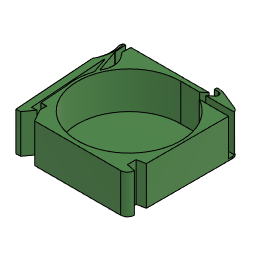
Compliant Strip Holder v3 (Autodesk Fusion 360 design; units mm, degrees)
Autodesk Fusion 360 part; units mm, degrees
sketch "Sketch1" plane through (0, 0, 0) normal (0, 0, 1) x (1, 0, 0) in component "Compliant SMD Magazine"
  line L0 (26.5, 5) -> (26.5, 10)
  line L1 (26.5, 10) -> (31.5, 11)
  line L2 (31.5, 4) -> (26.5, 5)
  line L3 (26.5, 7.5) -> (31.5, 7.5) construction
  line L4 (31.5, 4) -> (31.5, 0)
  line L5 (31.5, 0) -> (-22.4585, 0)
  line L6 (-22.4585, 0) -> (-26.5, 7)
  line L7 (-26.5, 7) -> (-26.5, 11)
  line L8 (-26.5, 11) -> (-31.5, 11)
  line L9 (31.5, 11) -> (31.5, 4) construction
  line L10 (31.5, 11) -> (31.5, 65)
  line L11 (31.5, 65) -> (-31.5, 65)
  circle A0 centre (0, 32.5) radius 30
  line L12 (0, 0) -> (0, 65) construction
  line L13 (-31.5, 65) -> (-31.5, 11)
  line L14 (30, 32.5) -> (-30, 32.5) construction
  line L15 (0, 1.75) -> (0, 22.5)
  point P0 (-30, 32.5)
  dimension "d28" = 5
  dimension "d29" = 7
  dimension "d30" = 58
  dimension "d31" = 4
  dimension "d32" = 4
  dimension "d34" = 120
  dimension "d36" = 11
  dimension "d37" = 5
  dimension "d38" = 54
  dimension "d39" = 60
  dimension "d43" = 1.5
  dimension "d44" = 1.5
  constraint midpoint L3.start L0
  constraint symmetric L1 L2 L3
  constraint vertical L4
  constraint perpendicular L4 L5
  constraint perpendicular L5 L7
  constraint perpendicular L7 L8
  constraint vertical L0
  constraint equal L1 L2
  constraint coincident L3.end L9
  constraint coincident L12.start L5
  constraint parallel L9 L10
  constraint perpendicular L10 L11
  constraint coincident L5 L12.start
  constraint coincident L11 L12.end
  constraint perpendicular L11 L12
  constraint midpoint A0.centre L12
  constraint vertical L13
  constraint coincident A0 L14.start
  constraint coincident A0 P0
  constraint horizontal L14
  constraint coincident A0.centre L14
  constraint coincident P0 L14.end
  constraint coincident A0.centre L15
  measures "d28" distance of L0.start L0.end
  measures "d29" distance of L2.start L1.end
  measures "d30" distance of L4 L7
  measures "d31" distance of L2.start L4.end
  measures "d32" distance of L6.end L7.end
  measures "d34" angle of L5 L6
  measures "d36" distance of L5 L8
  measures "d37" horizontal distance of L2.start L0.start
  measures "d38" distance of L1.end L10.end
  measures "d39" diameter of A0
  measures "d43" distance of L13 P0
  measures "d44" distance of L10 L14.start
extrude "Extrude1" add sketch "Sketch1" against normal blind 1 contours L0 L1 L2 L4 L5 L6 L7 L8 L10 L11 L13 | A0 makes body 1 in component "Compliant SMD Magazine"
extrude "Extrude2" add sketch "Sketch1" along normal blind 21.5 bodies 1 in component "Compliant SMD Magazine"
sketch "Sketch2" plane through (0, 0, 21.5) normal (0, 0, 1) x (-1, 0, 0) in component "Compliant SMD Magazine"
  circle A0 centre (0, -32.5) radius 30
  line L0 (-31.5, -11) -> (-31.5, -65)
  line L1 (-31.5, -65) -> (31.5, -65)
  line L2 (-14.5237, -58.75) -> (-31.5, -58.75)
  line L3 (0, -62.5) -> (-31.5, -62.5)
  line L4 (-10.996, -62.5) -> (-14, -65)
  line L5 (-14.496, -62.5) -> (-17.5, -65)
  dimension "d53" = 3.75
  dimension "d77" = 14
  dimension "d78" = 3.5
  constraint coincident A0 L2.start
  constraint coincident L0 L2.end
  constraint perpendicular L0 L2
  constraint coincident A0 L3.start
  constraint coincident L0 L3.end
  constraint perpendicular L0 L3
  constraint tangent A0 L3
  constraint coincident L3 L4.start
  constraint coincident L1 L4.end
  constraint coincident L3 L5.start
  constraint coincident L1 L5.end
  constraint parallel L4 L5
  measures "d53" distance of L2 L3
  measures "d77" distance of L0.end L5.end
  measures "d78" distance of L4.end L5.end
extrude "Extrude3" cut sketch "Sketch2" against normal blind 21.5 contours A0 L0 L2 L3 | L1 L3 L4 L5 bodies 1 in component "Compliant SMD Magazine"
fillet "Fillet1" radius 4 1 edges at (31.5, 65, 10.25) on bodies 1 in component "Compliant SMD Magazine"
sketch "Sketch3" plane through (0, 0, 21.5) normal (0, 0, 1) x (-1, 0, 0) in component "Compliant SMD Magazine"
  arc A0 (-31.2081, -62.5) -> (-27.5, -65) centre (-27.5, -61) ccw
  line L0 (-29.0157, -64.7017) -> (-16.8486, -69.6836)
  line L1 (-16.8486, -69.6836) -> (-13.8486, -69.6836)
  line L2 (-13.8486, -69.6836) -> (-13.8486, -68.1836)
  line L3 (-13.8486, -68.1836) -> (-16.3486, -68.1836)
  arc A1 (-17.5, -65) -> (-16.3486, -68.1836) centre (-16.3486, -66.3836) ccw
  line L4 (-14.496, -62.5) -> (-17.5, -65)
  line L5 (-27.5, -65) -> (-17.5, -65)
  point P0 (-17.5, -65)
  dimension "d73" = 1.8
  dimension "d74" = 3
  dimension "d75" = 2.5
  dimension "d76" = 1.5
  constraint coincident A0 L0.start
  constraint tangent A0 L0
  constraint horizontal L1
  constraint perpendicular L1 L2
  constraint perpendicular L2 L3
  constraint tangent L3 A1
  constraint coincident P0 A1.start
  constraint tangent A1 L4
  measures "d73" radius of A1
  measures "d74" distance of L0.end L1.end
  measures "d75" distance of L2.end L3.end
  measures "d76" distance of L1.end L2.end
extrude "Extrude4" add sketch "Sketch3" against normal blind 22.5 bodies 1 in component "Compliant SMD Magazine"
sketch "Sketch4" plane through (0, 0, 21.5) normal (0, 0, 1) x (-1, 0, 0) in component "Compliant SMD Magazine"
  arc A0 (0, -62.5) -> (-10.7703, -60.5) centre (0, -32.5) ccw
  line L0 (31.5, -65) -> (31.5, -11)
  line L1 (36.3782, -65.0029) -> (31.8329, -0.0029) construction
  line L2 (20.4207, -0.0029) -> (-27.5793, -0.0029)
  line L3 (-17.5793, -65.0029) -> (19.5511, -65.0029)
  circle A1 centre (0, -32.5) radius 31.5
  line L4 (31.5, -49) -> (35.2409, -48.7384) construction
  line L5 (38.3454, -64.4642) -> (33.8699, -0.462)
  line L6 (33.8699, -0.462) -> (31.2324, -0.6464)
  line L7 (31.2324, -0.6464) -> (27.2424, -6.1381)
  line L8 (27.2424, -6.1381) -> (30.2424, -5.9283)
  line L9 (30.2424, -5.9283) -> (34.3551, -64.7432)
  circle A2 centre (31.5, -49) radius 48.9982 construction
  circle A3 centre (31.5, -49) radius 16 construction
  line L10 (38.3454, -64.4642) -> (34.3551, -64.7432)
  line L11 (31.5, -11) -> (26.5, -11)
  line L12 (31.5, -11) -> (31.5, -65)
  line L13 (29.8452, -11) -> (31.5, -34.6644)
  arc A4 (41.7395, -45.8316) -> (43.1815, -72.1488) centre (53.9576, -58.3602) ccw
  line L14 (53.9576, -58.3602) -> (36.5003, -59.581) construction
  point P0 (31.5, -49)
  point P1 (31.8329, -0.0029)
  dimension "d81" = 16
  dimension "d84" = 4
  dimension "d85" = 1.5
  dimension "d87" = 3.75
  dimension "d88" = 4
  dimension "d89" = 3
  dimension "d90" = 5.2
  dimension "d92" = 130
  dimension "d95" = 0.6
  dimension "d96" = 0.75
  dimension "d109" = 35
  dimension "d110" = 5
  dimension "d112" = 1.5
  constraint coincident L0 P0
  constraint coincident P1 L2
  constraint coincident L1.start L3
  constraint concentric A0 A1
  constraint coincident P0 L4.start
  constraint coincident L1 L4.end
  constraint perpendicular L1 L4
  constraint perpendicular L1 L6
  constraint perpendicular L1 L8
  constraint perpendicular L8 L9
  constraint coincident L1 P1
  constraint coincident A2 P1
  constraint coincident P1 L1.end
  constraint coincident L0.start A3
  constraint coincident L9.end A3
  constraint perpendicular L5 L10
  constraint coincident L11 L13.start
  constraint coincident L0 L13.end
  constraint parallel L9 L13
  constraint coincident A4.centre L14.start
  constraint coincident L14.end A4
  constraint perpendicular L1 L14
  measures "d81" distance of L0.start P0
  measures "d84" angle of L0 L1
  measures "d85" distance of A0 A1
  measures "d87" distance of P0 L4.end
  measures "d88" distance of L5 L9
  measures "d89" horizontal distance of L7.end L8.end
  measures "d90" distance of L6 L8
  measures "d92" angle of L6 L7
  measures "d95" distance of P1 L6
  measures "d96" distance of L9 L13
  measures "d109" diameter of A4
  measures "d110" distance of L10 L14
  measures "d112" distance of L5 L14.end
extrude "Extrude5" cut sketch "Sketch4" against normal through all contours L0 A1 L9 L11 L12 L13 | L0 L9 L11 L12 bodies 1 in component "Compliant SMD Magazine"
extrude "Extrude6" add sketch "Sketch4" against normal blind 22.5 separate body contours L0 L9 L11 L12 | L0 L5 L6 L7 L8 L9 L10 L11 L12 A4 makes body 2 in component "Compliant SMD Magazine"
sketch "Sketch5" plane through (0, 0, 21.5) normal (0, 0, 1) x (-1, 0, 0) in component "Compliant SMD Magazine"
  circle A0 centre (0, -32.5) radius 31.5
  line L0 (30.2424, -5.9283) -> (34.3551, -64.7432) construction
  line L1 (31.5, -65) -> (31.5, -32.5) construction
  line L2 (29.1712, -44.3867) -> (33.89, -58.0911)
  line L3 (29.9351, -42.3051) -> (33.5127, -52.6951)
  line L4 (29.5632, -43.3751) -> (33.7013, -55.3931) construction
  line L5 (30.8587, -49.2877) -> (32.1824, -48.8319) construction
  line L6 (24.9005, -51.7929) -> (31.7944, -60.0087)
  line L7 (31.6323, -49.3841) -> (33.2424, -48.8297) construction
  line L8 (31.7944, -60.0087) -> (31.5, -65)
  line L9 (34.3551, -64.7432) -> (30.2424, -5.9283)
  line L10 (31.5, -32.5) -> (31.5, -65)
  line L11 (-14, -65) -> (31.5, -65)
  point P0 (31.5, -49)
  point P1 (32.4373, -49.1069)
  dimension "d100" = 15
  dimension "d101" = 1.4
  dimension "d117" = 5
  dimension "d118" = 50
  constraint coincident A0 L2.start
  constraint coincident L0 L2.end
  constraint coincident A0 L3.start
  constraint coincident L0 L3.end
  constraint coincident A0 L4.start
  constraint coincident L0 L4.end
  constraint coincident P0 L4
  constraint coincident L2 L5.start
  constraint coincident L3 L5.end
  constraint perpendicular L3 L5
  constraint parallel L3 L4
  constraint coincident A0 L6.start
  constraint coincident L4 L7.start
  constraint coincident L0 L7.end
  constraint perpendicular L4 L7
  constraint midpoint L4 L7.start
  constraint midpoint L7 P1
  constraint coincident L1.start L8.end
  constraint coincident P1 L8
  measures "d100" angle of L0 L4
  measures "d101" distance of L5.start L5.end
  measures "d117" distance of L6.end L1.start
  measures "d118" angle of L6 L11
extrude "Extrude7" cut sketch "Sketch5" against normal through all contours A0 L3 L10 | A0 L2 L6 L10 | A0 L2 L3 L10 bodies 1 in component "Compliant SMD Magazine"
extrude "Extrude8" add sketch "Sketch5" against normal blind 22.5 contours L6 L8 L10 bodies 1 in component "Compliant SMD Magazine"
extrude "Extrude9" add sketch "Sketch5" against normal blind 22.5 contours A0 L2 L3 L10 | L2 L3 L9 L10 bodies 1 2 in component "Compliant SMD Magazine"
chamfer "Chamfer1" distance 1.5 distance2 2 2 edges at (-36.458, 58.4681, 21.5) (-36.458, 58.4681, -1) measured on face at (-36.5666, 56.4106, 6.5) measured on face at (6.3665, 42.2643, -1) on bodies 1 in component "Compliant SMD Magazine"
fillet "Fillet2" radius 4 1 edges at (31.5, 0, 10.25) on bodies 1 in component "Compliant SMD Magazine"
fillet "Fillet3" radius 3 1 edges at (-31.7944, 60.0087, 10.25) on bodies 1 in component "Compliant SMD Magazine"
fillet "Fillet4" radius 11 1 edges at (-24.9005, 51.7929, 10.25) on bodies 1 in component "Compliant SMD Magazine"
fillet "Fillet5" radius 0.2 1 edges at (-33.5127, 52.6951, 10.25) on bodies 1 in component "Compliant SMD Magazine"
fillet "Fillet6" radius 0.25 1 edges at (-29.1712, 44.3867, 10.25) on bodies 1 in component "Compliant SMD Magazine"
fillet "Fillet7" radius 1.5 2 edges at (-29.9351, 42.3051, 10.25) (-33.89, 58.0911, 10.25) on bodies 1 in component "Compliant SMD Magazine"
fillet "Fillet8" radius 10 1 edges at (16.8486, 69.6836, 10.25) on bodies 1 in component "Compliant SMD Magazine"
scale "Scale1" factor 0.666667 about (-33.4067, 51.1797, 21.5) bodies 1 in component "Compliant SMD Magazine"
component "Compliant SMD Magazine" placed x (1, 0, 0) y (0, 1, 0) z (0, 0, 1) at (0, 0, 0)
equation "d47 = height - 1 mm"
equation "height = final_height / scale"
equation "d53 = gap_width"
equation "gap_width = final_gap_width / scale"
equation "d70 = -( height - 1 mm )"
equation "d79 = -height"
equation "d98 = -height"
equation "d101 = 1.4 mm * stiffness"
equation "d105 = -height"
equation "d107 = -height"
equation "stiffness = 1.0"
equation "scale = 2 / 3"
equation "final_height = 15 mm"
equation "final_gap_width = 2.5 mm"
equation "d138 = scale"
